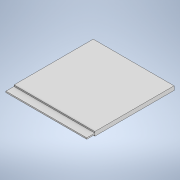
# Autodesk Inventor part: False_Bottom_3
Saved by Autodesk Inventor 2020 (Build 240168000, 168)
## iProperties
Created: 2022-01-22
Part Number: False_Bottom_3
Material: Generic
Document SubType Name: Modeling
Designer: danie
Density: 1 g/cm^3
Appearance: Default
Author: danie
Autodesk Inventor part; units mm, degrees
ref_plane "YZ Plane" through (0, 0, 0) normal (1, 0, 0) x (0, 1, 0)
ref_plane "XZ Plane" through (0, 0, 0) normal (0, 1, 0) x (-1, 0, 0)
ref_plane "XY Plane" through (0, 0, 0) normal (0, 0, 1) x (1, 0, 0)
sketch "Sketch1" plane through (0, 0, 0) normal (0, 1, 0) x (-1, 0, 0)
  line L0 (0, 0) -> (-127, 0)
  line L1 (-127, 0) -> (-127, -124.46)
  line L2 (-127, -124.46) -> (0, -124.46)
  line L3 (0, -124.46) -> (0, 0)
  dimension "d0" = 127
  dimension "d1" = 124.46
  constraints: 8 end point, 2 parallel, 1 horizontal, 1 perpendicular
  measures "d0" distance of L2.end L1.end
  measures "d1" distance of L1.end L0.end
extrude "Extrusion1" add sketch "Sketch1" along normal blind 6.35
sketch "Sketch2" plane through (0, 0, 0) normal (0, 0, 1) x (1, 0, 0)
  line L0 (0, 6.35) -> (127, 6.35) construction
  line L1 (0, 6.35) -> (2.921, 6.35) construction
  line L2 (0, 0) -> (127, 0) construction
  line L3 (127, 3.429) -> (127, 2.921) construction
  line L4 (0, 6.35) -> (0, 4.191) construction
  line L5 (0, 0) -> (0, 6.35) construction
  line L6 (0, 6.35) -> (2.159, 6.35) construction
  line L7 (0, 0) -> (0, 2.159) construction
  line L8 (0, 4.191) -> (0, 2.159)
  line L9 (0, 2.159) -> (127, 2.159)
  line L10 (127, 2.159) -> (127, 4.191)
  line L11 (127, 4.191) -> (0, 4.191)
  dimension "d9" = 2.159
  dimension "d10" = 90
  dimension "d11" = 2.159
  constraints: 18 end point, 2 collinear, 2 horizontal, 2 parallel, 2 perpendicular, 1 point on line
  measures "d9" distance of L0.start L4.end
  measures "d10" angle of L4 L6
  measures "d11" distance of L2.start L7.end
extrude "Extrusion2" add sketch "Sketch2" along normal blind 12.7
body "Solid1"
